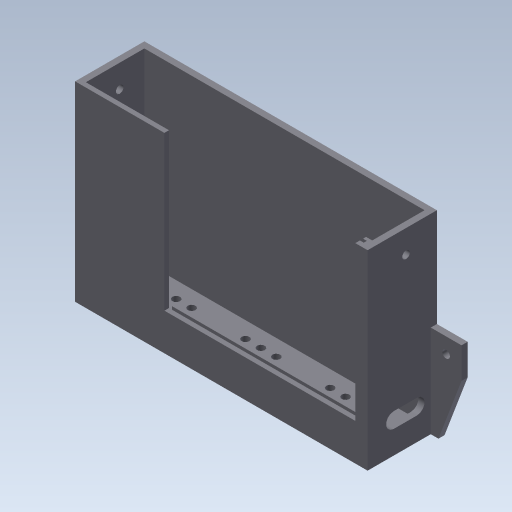
# Autodesk Inventor part: krab2-ver1
Saved by Autodesk Inventor 2023 (Build 270158000, 158)
## iProperties
Created: 2024-03-18
Part Number: krab2-ver1
Material: 11 500
Document SubType Name: Modeling
Designer: sok
Density: 7.86 g/cm^3
Appearance: Kov-Ocel
Author: sok
Autodesk Inventor part; units mm, degrees
ref_plane "YZ Plane" through (0, 0, 0) normal (1, 0, 0) x (0, 1, 0)
ref_plane "XZ Plane" through (0, 0, 0) normal (0, 1, 0) x (-1, 0, 0)
ref_plane "XY Plane" through (0, 0, 0) normal (0, 0, 1) x (1, 0, 0)
sketch "Náčrt2" plane through (0, 0, 0) normal (0, 0, 1) x (1, 0, 0)
  line L0 (0, 0) -> (190, 0)
  line L1 (190, 0) -> (190, -45)
  line L2 (190, -45) -> (0, -45)
  line L3 (0, -45) -> (0, 0)
  dimension "d2" = 190
  dimension "d3" = 45
  constraints: 8 end point, 2 parallel, 1 horizontal, 1 perpendicular
  measures "d2" distance of L1.end L2.end
  measures "d3" distance of L0.end L1.end
extrude "Vysunutí2" add sketch "Náčrt2" along normal blind 4
sketch "Náčrt3" plane through (0, 0, 4) normal (0, 0, 1) x (1, 0, 0)
  line L0 (190, 0) -> (0, 0) projected
  line L1 (0, -45) -> (190, -45) projected
  line L2 (190, -45) -> (190, 0) projected
  line L3 (190, 0) -> (0, 0) projected
  line L4 (0, 0) -> (0, -45) projected
  line L5 (4, -41) -> (186, -41)
  line L6 (186, -41) -> (186, -4)
  line L7 (186, -4) -> (4, -4)
  line L8 (4, -4) -> (4, -41)
  dimension "d7" = 4
  constraints: 8 end point, 3 other
  measures "d7" distance between parallel lines of L4 L8
extrude "Vysunutí3" add sketch "Náčrt3" along normal blind 120
sketch "Náčrt4" plane through (0, -45, 0) normal (0, -1, 0) x (1, 0, 0)
  line L0 (4, 124) -> (186, 124) projected
  line L1 (182, 124) -> (58, 124)
  line L2 (58, 124) -> (58, 24)
  line L3 (58, 24) -> (182, 24)
  line L4 (182, 24) -> (182, 124)
  line L5 (190, 0) -> (190, 124) projected
  point P0 (0, 0)
  dimension "d10" = 8
  dimension "d11" = 100
  dimension "d12" = 124
  constraints: 8 end point, 2 parallel, 1 horizontal, 1 perpendicular, 1 point on line
  measures "d10" distance between parallel lines of L5 L4
  measures "d11" distance of L3.end L1.start
  measures "d12" distance of L2.end L3.end
extrude "Vysunutí4" cut sketch "Náčrt4" against normal blind 10
sketch "Náčrt6" plane through (4, -41, 4) normal (0, 1, 0) x (1, 0, 0)
  line L0 (-4, 4) -> (186, 4) projected
  line L1 (-4, 4) -> (-4, -120) projected
  line L2 (178, -120) -> (178, -20) projected
  line L3 (178, -20) -> (54, -20) projected
  line L4 (54, -20) -> (54, -120) projected
  line L5 (-4, -120) -> (54, -120) projected
  line L6 (-4, 4) -> (-4, -120) projected
  line L7 (-4, 4) -> (186, 4) projected
  line L8 (186, 4) -> (186, -120) projected
  line L9 (178, -120) -> (186, -120) projected
extrude "Vysunutí6" add sketch "Náčrt6" along normal blind 3
sketch "Náčrt7" plane through (0, 0, 124) normal (0, 0, 1) x (1, 0, 0)
  line L0 (184.5, -42) -> (4, -42)
  line L1 (4, -42) -> (4, -40)
  line L2 (4, -40) -> (184.5, -40)
  line L3 (184.5, -40) -> (184.5, -42)
  line L4 (182, -38) -> (182, -45) projected
  line L5 (182, -45) -> (190, -45) projected
  point P0 (0, 0)
  dimension "d25" = 2.5
  dimension "d26" = 2
  dimension "d27" = 3
  dimension "d28" = 180.5
  constraints: 8 end point, 2 parallel, 1 horizontal, 1 perpendicular
  measures "d25" distance between parallel lines of L3 L4
  measures "d26" distance of L2.end L0.start
  measures "d27" distance between parallel lines of L5 L0
  measures "d28" distance of L0.start L0.end
extrude "Vysunutí7" cut sketch "Náčrt7" against normal blind 105
sketch "Náčrt8" plane through (4, -38, 4) normal (0, 1, 0) x (1, 0, 0)
  line L0 (54, -120) -> (54, -20) projected
  line L1 (0, -120) -> (54, -120) projected
  line L2 (54, -120) -> (0, -120)
  line L3 (0, -120) -> (0, -20)
  line L4 (0, -20) -> (54, -20)
  line L5 (54, -20) -> (54, -120)
  point P0 (-4, 4)
  point P1 (54, -20)
  dimension "d31" = 54
  dimension "d32" = 100
  constraints: 8 end point, 2 parallel, 1 horizontal, 1 perpendicular
  measures "d31" distance of L3.end L4.end
  measures "d32" distance between parallel lines of L1 L4
extrude "Vysunutí8" cut sketch "Náčrt8" against normal up to surface (4 mm away)
sketch "Náčrt9" plane through (4, -38, 4) normal (0, 1, 0) x (1, 0, 0)
  line L0 (54, -20) -> (54, -120) projected
  line L1 (0, 40) -> (54, 40)
  line L2 (54, 40) -> (54, -20)
  line L3 (54, -20) -> (0, -20)
  line L4 (0, -20) -> (0, 40)
  point P0 (-4, 4)
  dimension "d35" = 54
  constraints: 8 end point, 2 parallel, 1 horizontal, 1 perpendicular
  measures "d35" distance of L1.start L1.end
extrude "Vysunutí9" cut sketch "Náčrt9" against normal blind 4
sketch "Náčrt10" plane through (190, -45, 0) normal (1, 0, 0) x (0, 0, -1)
  circle A0 centre (-109, 25) radius 2.5
  line L0 (0, 0) -> (-124, 0) projected
  line L1 (-124, 0) -> (-124, 45) projected
  point P0 (0, 45)
  dimension "d38" = 5
  dimension "d39" = 25
  dimension "d40" = 15
  constraints: 1 centre point
  measures "d38" diameter of A0
  measures "d39" distance from line of A0.centre L0
  measures "d40" distance from line of A0.centre L1
extrude "Vysunutí10" cut sketch "Náčrt10" against normal through all
sketch "Náčrt11" plane through (0, 0, 4) normal (0, 0, 1) x (1, 0, 0)
  circle A0 centre (25.2842, -14.6015) radius 2.5
  circle A1 centre (35.2842, -14.6015) radius 2.5
  circle A2 centre (45.2842, -14.6015) radius 2.5
  circle A3 centre (31.1056, -24.6015) radius 2.5
  circle A4 centre (41.1056, -24.6015) radius 2.5
  circle A5 centre (36.7049, -34.6015) radius 2.5
  line L0 (25.2842, -14.6015) -> (59.2692, -14.6015) construction
  line L1 (31.1056, -24.6015) -> (52.5835, -24.6015) construction
  point P0 (0, 0)
  dimension "d43" = 5
  dimension "d44" = 5
  dimension "d45" = 5
  dimension "d46" = 5
  dimension "d47" = 5
  dimension "d48" = 5
  dimension "d49" = 10
  dimension "d50" = 10
  dimension "d51" = 10
  dimension "d52" = 10
  dimension "d53" = 10
  constraints: 6 centre point, 4 end point, 3 point on line, 2 horizontal
  measures "d43" diameter of A0
  measures "d44" diameter of A1
  measures "d45" diameter of A2
  measures "d46" diameter of A3
  measures "d47" diameter of A4
  measures "d48" diameter of A5
  measures "d49" distance of A1.centre L0.start
  measures "d50" distance of A2.centre A1.centre
  measures "d51" distance of A4.centre L1.start
  measures "d52" distance between parallel lines of L1 L0
  measures "d53" distance from line of A5.centre L1
extrude "Vysunutí11" cut sketch "Náčrt11" against normal through all
pattern_linear "Obdélníkové pole1" count 3 spacing 55 along (1, 0, 0) of "Vysunutí11"
sketch "Náčrt12" plane through (0, 0, 0) normal (0, 0, -1) x (-1, 0, 0)
  line L0 (-4, -42) -> (-58, -42) projected
  line L1 (-58, -38) -> (-4, -38) projected
  line L2 (-58, -42) -> (-58, -38) projected
  line L3 (-4, -38) -> (-4, -42) projected
  point P0 (0, 0)
extrude "Vysunutí12" add sketch "Náčrt12" against normal up to surface (4 mm away)
sketch "Náčrt13" plane through (190, -45, 0) normal (1, 0, 0) x (0, 0, -1)
  line L0 (-20, 12) -> (-20, 37) construction
  line L1 (-15, 17) -> (-15, 32)
  line L2 (-25, 32) -> (-25, 17)
  arc A0 (-25, 17) -> (-15, 17) centre (-20, 17) ccw
  arc A1 (-15, 32) -> (-25, 32) centre (-20, 32) ccw
  line L3 (0, 45) -> (-124, 45) projected
  line L4 (0, 0) -> (0, 45) projected
  point P0 (-20, 24.5)
  dimension "d61" = 25
  dimension "d62" = 10
  dimension "d63" = 8
  dimension "d64" = 20
  constraints: 8 end point, 6 point on circle, 4 tangent, 2 centre point, 2 point on line, 1 midpoint, 1 parallel, 1 vertical
  measures "d61" distance of L0.start L0.end
  measures "d62" diameter of A1
  measures "d63" distance from line of L3 L0.end
  measures "d64" distance between parallel lines of L4 L0
extrude "Vysunutí13" cut sketch "Náčrt13" against normal through all
sketch "Náčrt14" plane through (0, 0, 0) normal (0, 1, 0) x (1, 0, 0)
  line L0 (190, 0) -> (190, -124) projected
  line L1 (190, -60) -> (210, -60)
  line L2 (210, -60) -> (210, -40)
  line L3 (210, -40) -> (190, -40)
  line L4 (190, -40) -> (190, -60)
  line L5 (190, 0) -> (0, 0) projected
  line L6 (190, 0) -> (195, 0)
  line L7 (195, 0) -> (210, -40)
  circle A0 centre (200, -50) radius 2.5
  line L8 (4, -124) -> (186, -124) projected
  line L9 (95, -124) -> (95, 0) construction
  line L10 (0, 0) -> (0, -124)
  line L11 (0, -60) -> (-20, -60)
  line L12 (-20, -60) -> (-20, -40)
  line L13 (-20, -40) -> (0, -40)
  line L14 (0, 0) -> (190, 0)
  line L15 (0, 0) -> (-5, 0)
  line L16 (-5, 0) -> (-20, -40)
  circle A1 centre (-10, -50) radius 2.5
  dimension "d67" = 20
  dimension "d68" = 20
  dimension "d69" = 40
  dimension "d70" = 5
  dimension "d71" = 5
  dimension "d72" = 10
  dimension "d73" = 10
  constraints: 28 end point, 9 symmetric about line, 2 centre point, 2 horizontal, 2 midpoint, 2 parallel, 2 point on line, 1 perpendicular, 1 other
  measures "d67" distance of L3.end L2.end
  measures "d68" distance of L1.end L2.end
  measures "d69" distance between parallel lines of L5 L3
  measures "d70" distance of L0.start L6.end
  measures "d71" diameter of A0
  measures "d72" distance from line of L2 A0.centre
  measures "d73" distance from line of A0.centre L1
extrude "Vysunutí14" add sketch "Náčrt14" against normal blind 4
